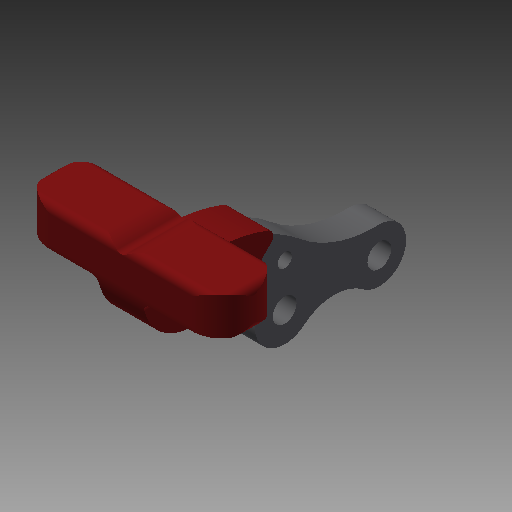
# Autodesk Inventor part: 305104_105
Saved by Autodesk Inventor 2018 (Build 220112000, 112)
## iProperties
Category: PARTsolutions
Company: DESTACO
Created: 2018-01-28
Part Number: 305104_105
Catalog Web Link: www.cadenas.de
Description: 305104_105-Zwischenstuck
Vendor: DESTACO
Document SubType Name: Modeling
Designer: psAdmin
Manufacturer: DESTACO
Mass: 2.27971 g
Surface Area: 16.7149 cm^2
Volume: 2.27971 cm^3
Density: 1 g/cm^3
Material: Generic
Appearance: PSOLRGB-192-192-192
PSOL_IDENT_0: {$CADENAS_DATA\23d-libs\destaco\destaco_gmbh\man_spann\horizontalspanner\kompaktspan_mit_zusat\305ur
PSOL_IDENT_1: _bis_309ur_parts\handgriff_ur.prj},159 {VTYP=3D},{NB=305104_105},{LINA=305104_105},{NN=305104_105},{
PSOL_IDENT_2: DATE=20.09.2016 07:53:11},{GEOMDATE=27.06.2006},{VERSION=v1},{LINEID=10},{LINESUBID=-1},{WBVAR=}  {N
PSOL_IDENT_3: B=305104_105},{LINA=305104_105},{KT=DUMMY},{MODELL=305104_105},{SIZE=1.000}
NN: 305104_105
NT: Zwischenstuck
NB: 305104_105
NBSYN: $MODELL.
LINA: 305104_105
MODELL: 305104_105
SIZE: 1.000
SUPPLIER: DESTACO
ARTICLENO: 305104_105
BOMINFO: 305104_105
CREATOR: CADENAS GmbH
Title: 305104_105
Author: Cadenas PARTsolutions
Comments: Zwischenstuck
Autodesk Inventor part; units mm, degrees
sketch "Skizze_4" plane through (0, 0, 0) normal (1, 0, 0) x (0, 1, 0)
  line L0 (14.3, 31.7) -> (11.8, 31.7)
  arc A0 (11.8, 31.7) -> (6.3, 26.2) centre (11.8, 26.2) ccw
  line L1 (6.3, 26.2) -> (6.3, 23)
  arc A1 (0, 16.7) -> (6.3, 23) centre (0, 23) ccw
  arc A2 (0, 16.7) -> (-3.0486, 10.1104) centre (0, 12.7) ccw
  arc A3 (-2.8546, 2.1934) -> (-3.0486, 10.1104) centre (-7.8502, 6.0319) ccw
  arc A4 (-2.8546, 2.1934) -> (3.5986, 0.1012) centre (0, 0) ccw
  arc A5 (7.1983, 10.6002) -> (3.5986, 0.1012) centre (19.3921, 0.5528) ccw
  arc A6 (7.1983, 10.6002) -> (11.8856, 24.4701) centre (-8.7, 23.7) ccw
  arc A7 (12.685, 25.3) -> (11.8856, 24.4701) centre (12.685, 24.5) ccw
  line L2 (12.685, 25.3) -> (14.3, 25.3)
  line L3 (14.3, 25.3) -> (14.3, 31.7)
  circle A8 centre (5.8, 12.7) radius 0.965
  constraints: 16 point on circle, 9 centre point, 8 end point
extrude "Extrusion1" add sketch "Skizze_4" along normal mid plane 4
sketch "Sketch_1" plane through (0, 0, 0) normal (1, 0, 0) x (0, 1, 0)
  line L0 (14.3, 32.7) -> (11.8, 32.7)
  arc A0 (11.8, 32.7) -> (5.3, 26.2) centre (11.8, 26.2) ccw
  line L1 (5.3, 26.2) -> (5.3, 23)
  arc A1 (4.9518, 21.1105) -> (5.3, 23) centre (0, 23) ccw
  arc A2 (4.9518, 21.1105) -> (5.1789, 20.0469) centre (5.8861, 20.754) ccw
  line L2 (5.1789, 20.0469) -> (9.6942, 15.5317)
  arc A3 (9.6942, 15.5317) -> (11.3334, 15.8766) centre (10.4013, 16.2388) ccw
  arc A4 (11.3334, 15.8766) -> (12.7966, 23.3177) centre (-8.8, 23.7) ccw
  arc A5 (13.7965, 24.3) -> (12.7966, 23.3177) centre (13.7965, 23.3) ccw
  line L3 (13.7965, 24.3) -> (14.3, 24.3)
  arc A6 (14.3, 24.3) -> (15.3, 25.3) centre (14.3, 25.3) ccw
  line L4 (15.3, 25.3) -> (15.3, 31.7)
  arc A7 (15.3, 31.7) -> (14.3, 32.7) centre (14.3, 31.7) ccw
  constraints: 16 point on circle, 10 end point, 8 centre point
extrude "Extrusion2" add sketch "Sketch_1" along normal mid plane 6
sketch "Skizze_5_ALT_Drilling_1" plane through (0, 0, 0) normal (0, 1, 0) x (-1, 0, 0)
  line L0 (10, 0) -> (-10, 0)
  line L1 (-10, 0) -> (-10, 1.6)
  line L2 (-10, 1.6) -> (10, 1.6)
  line L3 (10, 1.6) -> (10, 0)
  line L4 (10, 0) -> (-10, 0)
  constraints: 10 end point
revolve "Revolution1" cut sketch "Skizze_5_ALT_Drilling_1" angle 360 about axis through (-10, 0, 0) along (-1, 0, 0)
sketch "Skizze_6_ALT_Drilling_2" plane through (0, 0, 0) normal (0, 1, 0) x (-1, 0, 0)
  line L0 (10, 12.7) -> (-10, 12.7)
  line L1 (-10, 12.7) -> (-10, 14.3)
  line L2 (-10, 14.3) -> (10, 14.3)
  line L3 (10, 14.3) -> (10, 12.7)
  line L4 (10, 12.7) -> (-10, 12.7)
  constraints: 10 end point
revolve "Revolution2" cut sketch "Skizze_6_ALT_Drilling_2" angle 360 about axis through (-10, 0, 12.7) along (-1, 0, 0)
sketch "Sketch_2" plane through (0, 16.4, 0) normal (0, 1, 0) x (1, 0, 0)
  arc A0 (-9.5, -24.3) -> (-9.5, -32.7) centre (-9.5, -28.5) ccw
  line L0 (-9.5, -32.7) -> (9.5, -32.7)
  arc A1 (9.5, -32.7) -> (9.5, -24.3) centre (9.5, -28.5) ccw
  line L1 (9.5, -24.3) -> (-9.5, -24.3)
  constraints: 4 end point, 4 point on circle, 2 centre point
extrude "Extrusion3" add sketch "Sketch_2" against normal blind 6.1
sketch "Sketch_3" plane through (0, 0, 0) normal (1, 0, 0) x (0, 1, 0)
  line L0 (-12.0571, 36.1801) -> (-12.0571, -15.6384)
  line L1 (-12.0571, -15.6384) -> (20.4908, -15.6384)
  line L2 (20.4908, -15.6384) -> (20.4908, 36.1801)
  line L3 (20.4908, 36.1801) -> (-12.0571, 36.1801)
  line L4 (15.4, 32.7) -> (11.8, 32.7)
  arc A0 (11.8, 32.7) -> (5.3, 26.2) centre (11.8, 26.2) ccw
  line L5 (5.3, 26.2) -> (-6.4975, 26.2)
  line L6 (-6.4975, 26.2) -> (-6.4975, -9.3)
  line L7 (-6.4975, -9.3) -> (15.4, -9.3)
  line L8 (15.4, -9.3) -> (15.4, 24.3)
  arc A1 (15.4, 24.3) -> (16.4, 25.3) centre (15.4, 25.3) ccw
  line L9 (16.4, 25.3) -> (16.4, 31.7)
  arc A2 (16.4, 31.7) -> (15.4, 32.7) centre (15.4, 31.7) ccw
  constraints: 20 end point, 6 point on circle, 3 centre point
extrude "Extrusion4" cut sketch "Sketch_3" along normal mid plane 40
sketch "Sketch_4" plane through (0, 0, 32.7) normal (0, 0, 1) x (1, 0, 0)
  line L0 (-22.6525, -16.2217) -> (-3, -16.2217)
  line L1 (-3, -16.2217) -> (-3, 10.3)
  arc A0 (-3, 10.3) -> (-4, 11.3) centre (-4, 10.3) ccw
  line L2 (-4, 11.3) -> (-12.7, 11.3)
  arc A1 (-13.7, 12.3) -> (-12.7, 11.3) centre (-12.7, 12.3) ccw
  line L3 (-13.7, 12.3) -> (-13.7, 15.4)
  arc A2 (-12.7, 16.4) -> (-13.7, 15.4) centre (-12.7, 15.4) ccw
  line L4 (-12.7, 16.4) -> (-2.7982, 16.4)
  arc A3 (-0.583, 15.6875) -> (-2.7982, 16.4) centre (-2.7982, 12.6) ccw
  arc A4 (-0.583, 15.6875) -> (0.583, 15.6875) centre (0, 16.5) ccw
  arc A5 (2.7982, 16.4) -> (0.583, 15.6875) centre (2.7982, 12.6) ccw
  line L5 (2.7982, 16.4) -> (12.7, 16.4)
  arc A6 (13.7, 15.4) -> (12.7, 16.4) centre (12.7, 15.4) ccw
  line L6 (13.7, 15.4) -> (13.7, 12.3)
  arc A7 (12.7, 11.3) -> (13.7, 12.3) centre (12.7, 12.3) ccw
  line L7 (12.7, 11.3) -> (4, 11.3)
  arc A8 (4, 11.3) -> (3, 10.3) centre (4, 10.3) ccw
  line L8 (3, 10.3) -> (3, -16.2217)
  line L9 (3, -16.2217) -> (21.2638, -16.2217)
  line L10 (21.2638, -16.2217) -> (21.2638, 23.8758)
  line L11 (21.2638, 23.8758) -> (-22.6525, 23.8758)
  line L12 (-22.6525, 23.8758) -> (-22.6525, -16.2217)
  constraints: 26 end point, 18 point on circle, 9 centre point
extrude "Extrusion5" cut sketch "Sketch_4" against normal blind 10
ref_plane "HG1_XY" through (0, 0, 0) normal (1, 0, 0) x (0, 0, -1)
ref_plane "HG1_YZ" through (0, 0, 0) normal (0, 0, -1) x (0, 1, 0)
ref_plane "HG1_ZX" through (0, 0, 0) normal (0, 1, 0) x (1, 0, 0)
ref_plane "HG2_XY" through (0, 0, 12.7) normal (1, 0, 0) x (0, 0, -1)
ref_plane "HG2_YZ" through (0, 0, 12.7) normal (0, 0, -1) x (0, 1, 0)
ref_plane "HG2_ZX" through (0, 0, 12.7) normal (0, 1, 0) x (1, 0, 0)
ref_plane "HG3_XY" through (0, 0, 0) normal (0, 0, 1) x (1, 0, 0)
ref_plane "HG3_YZ" through (0, 0, 0) normal (1, 0, 0) x (0, 1, 0)
ref_plane "HG3_ZX" through (0, 0, 0) normal (0, 1, 0) x (0, 0, 1)
body "Solid1"
